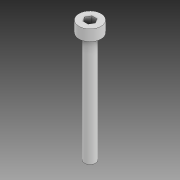
# Autodesk Inventor part: M3x30 SHCS
Saved by Autodesk Inventor 2020 (Build 240168000, 168)
## iProperties
Created: 2021-05-21
Part Number: M3x30 SHCS
Material: Generic
Document SubType Name: Modeling
Designer: DDeGo
Density: 1 g/cm^3
Appearance: Default
Author: DDeGo
Autodesk Inventor part; units mm, degrees
ref_plane "YZ Plane" through (0, 0, 0) normal (1, 0, 0) x (0, 1, 0)
ref_plane "XZ Plane" through (0, 0, 0) normal (0, 1, 0) x (-1, 0, 0)
ref_plane "XY Plane" through (0, 0, 0) normal (0, 0, 1) x (1, 0, 0)
sketch "Sketch1" plane through (0, 0, 0) normal (0, 0, 1) x (1, 0, 0)
  line L0 (0, 0) -> (0, 33)
  line L1 (0, 33) -> (3, 33)
  line L2 (3, 33) -> (3, 30)
  line L3 (3, 30) -> (1.5, 30)
  line L4 (1.5, 30) -> (1.5, 0)
  line L5 (1.5, 0) -> (0, 0)
  dimension "d0" = 30
  dimension "d1" = 1.5
  dimension "d2" = 3
  dimension "d3" = 3
  constraints: 12 end point, 5 perpendicular, 1 vertical
  measures "d0" distance between parallel lines of L5 L3
  measures "d1" distance between parallel lines of L4 L0
  measures "d2" distance between parallel lines of L0 L2
  measures "d3" distance of L1.end L2.end
revolve "Revolution1" add sketch "Sketch1" angle 360 about axis through (0, 0, 0) along (0, 1, 0)
sketch "Sketch2" plane through (0, 33, 0) normal (0, 1, 0) x (1, 0, 0)
  line L0 (0.7217, 1.25) -> (1.4434, 0)
  line L1 (1.4434, 0) -> (0.7217, -1.25)
  line L2 (0.7217, -1.25) -> (-0.7217, -1.25)
  line L3 (-0.7217, -1.25) -> (-1.4434, 0)
  line L4 (-1.4434, 0) -> (-0.7217, 1.25)
  line L5 (-0.7217, 1.25) -> (0.7217, 1.25)
  point P0 (0, 0)
  point P1 (0, 0)
  dimension "d5" = 2.5
  constraints: 12 end point, 1 coincident, 1 horizontal, 13 other
  measures "d5" distance between parallel lines of L1 L4
extrude "Extrusion1" cut sketch "Sketch2" against normal blind 3
body "Solid1"
